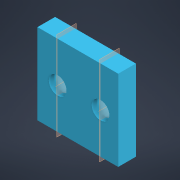
# Autodesk Inventor part: Parte 6
Saved by Autodesk Inventor 2021 (Build 250183000, 183)
## iProperties
Created: 2020-10-13
Part Number: Parte 6
Material: Steel, Galvanized
Document SubType Name: Modeling
Designer: Esteban
Density: 7.85 g/cm^3
Appearance: Turquoise
Author: Esteban
Autodesk Inventor part; units mm, degrees
ref_plane "YZ Plane" through (0, 0, 0) normal (1, 0, 0) x (0, 1, 0)
ref_plane "XZ Plane" through (0, 0, 0) normal (0, 1, 0) x (-1, 0, 0)
ref_plane "XY Plane" through (0, 0, 0) normal (0, 0, 1) x (1, 0, 0)
sketch "Sketch1" plane through (0, 0, 0) normal (0, 0, 1) x (1, 0, 0)
  line L0 (-16, -16) -> (16, -16)
  line L1 (16, -16) -> (16, 16)
  line L2 (16, 16) -> (-16, 16)
  line L3 (-16, 16) -> (-16, -16)
  line L4 (-16, -16) -> (16, 16) construction
  line L5 (16, -16) -> (-16, 16) construction
  circle A0 centre (-8, 0) radius 3.1981 construction
  point P0 (0, 0)
  dimension "d0" = 32
  dimension "d1" = 32
  dimension "d3" = 8
  constraints: 12 end point, 2 midpoint, 2 parallel, 1 centre point, 1 horizontal, 1 perpendicular
  measures "d0" distance of L0.start L0.end
  measures "d1" distance of L1.end L0.end
  measures "d3" distance from line of L3 A0.centre
extrude "Extrusion1" add sketch "Sketch1" along normal blind 7
sketch "Sketch2" plane through (0, 0, 7) normal (0, 0, 1) x (1, 0, 0)
  circle A0 centre (-8, 0) radius 3.5
  line L0 (-16, 16) -> (-16, -16) projected
  circle A1 centre (9, 0) radius 3.5
  line L1 (16, -16) -> (16, 16) projected
  point P0 (0, 0)
  dimension "d6" = 7
  dimension "d7" = 8
  dimension "d8" = 7
  dimension "d9" = 7
  constraints: 2 centre point
  measures "d6" diameter of A0
  measures "d7" distance from line of L0 A0.centre
  measures "d8" diameter of A1
  measures "d9" distance from line of L1 A1.centre
extrude "Extrusion2" cut sketch "Sketch2" against normal blind 7
ref_plane "Work Plane1" through (9, 0, 7) normal (1, 0, 0) x (0, 0, -1)
sketch "Sketch3" plane through (9, 0, 7) normal (1, 0, 0) x (0, 0, -1)
  line L0 (0, 3.5) -> (7, 3.5) construction
  line L1 (0, 3.5) -> (2, 3.5) construction
  line L2 (2, 3.5) -> (2, -3.5)
  line L3 (0, -3.5) -> (7, -3.5) projected
  line L4 (2, -3.5) -> (7, -6.3868)
  line L5 (2, -3.5) -> (7.7735, -3.5) construction
  line L6 (2, 3.5) -> (7, 6.3868)
  line L7 (7, 16) -> (7, -16) projected
  line L8 (2, 3.5) -> (7.7735, 3.5) construction
  line L9 (7, 6.3868) -> (7, -6.3868)
  line L10 (-1.5547, 0) -> (9.3282, 0) projected
  point P0 (7, 0)
  dimension "d13" = 2
  dimension "d14" = 30
  dimension "d15" = 30
  constraints: 14 end point, 4 point on line, 2 equal length, 2 horizontal, 2 vertical
  measures "d13" distance of L1.start L1.end
  measures "d14" angle of L4 L5
  measures "d15" angle of L8 L6
revolve "Revolution1" cut sketch "Sketch3" angle 360 about axis through (9, 0, 7) along (0, 0, -1) contours L3 L7 L4
ref_plane "Work Plane2" through (-8, 0, 7) normal (1, 0, 0) x (0, 0, -1)
sketch "Sketch4" plane through (-8, 0, 7) normal (1, 0, 0) x (0, 0, -1)
  line L0 (7, -6.3868) -> (2, -3.5) projected
  line L1 (2, -3.5) -> (7, -6.3868)
  line L2 (7, 16) -> (7, -16) projected
  line L3 (7, -3.5) -> (2, -3.5)
  line L4 (-1.4, 0) -> (8.4, 0) projected
  point P0 (7, 0)
  constraints: 4 end point, 3 point on line, 1 perpendicular
revolve "Revolution2" cut sketch "Sketch4" angle 360 about axis through (-8, 0, 7) along (0, 0, -1)
body "Solid1"
